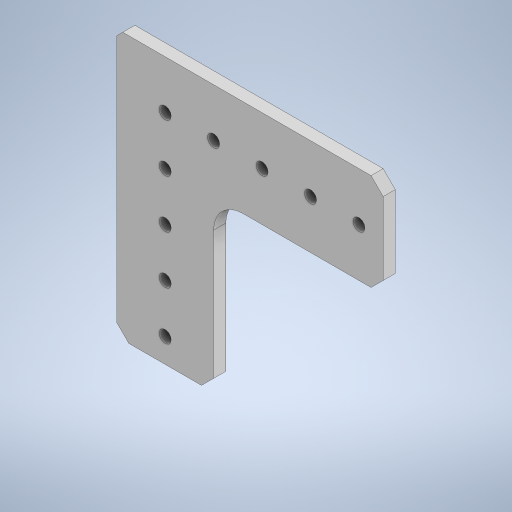
# Autodesk Inventor part: L-Bracket
Saved by Autodesk Inventor 2023 (Build 270158030, 158C)
## iProperties
Created: 2022-07-21
Part Number: L-Bracket
Material: Generic
Document SubType Name: Modeling
Designer: rm0990889
Density: 1 g/cm^3
Appearance: Default
Author: rm0990889
Autodesk Inventor part; units mm, degrees
ref_plane "YZ Plane" through (0, 0, 0) normal (1, 0, 0) x (0, 1, 0)
ref_plane "XZ Plane" through (0, 0, 0) normal (0, 1, 0) x (-1, 0, 0)
ref_plane "XY Plane" through (0, 0, 0) normal (0, 0, 1) x (1, 0, 0)
sketch "Sketch1" plane through (0, 0, 0) normal (0, 0, 1) x (1, 0, 0)
  circle A0 centre (12.7, -12.7) radius 1.5875
  line L0 (0, 0) -> (0, -14.9496)
  line L1 (0, 0) -> (27.0799, 0)
  circle A1 centre (25.4, -12.7) radius 1.5875
  circle A2 centre (38.1, -12.7) radius 1.5875
  circle A3 centre (50.8, -12.7) radius 1.5875
  circle A4 centre (63.5, -12.7) radius 1.5875
  circle A5 centre (12.7, -25.4) radius 1.5875
  circle A6 centre (12.7, -38.1) radius 1.5875
  circle A7 centre (12.7, -50.8) radius 1.5875
  circle A8 centre (12.7, -63.5) radius 1.5875
  line L2 (27.0799, 0) -> (66.675, 0)
  line L3 (69.85, -3.175) -> (69.85, -22.225)
  line L4 (0, -14.9496) -> (0, -66.675)
  line L5 (3.175, -69.85) -> (22.225, -69.85)
  line L6 (66.675, -25.4) -> (33.02, -25.4)
  line L7 (25.4, -33.02) -> (25.4, -66.675)
  arc A9 (33.02, -25.4) -> (25.4, -33.02) centre (33.02, -33.02) ccw
  line L8 (66.675, 0) -> (69.85, -3.175)
  line L9 (66.675, -25.4) -> (69.85, -22.225)
  line L10 (0, -66.675) -> (3.175, -69.85)
  line L11 (22.225, -69.85) -> (25.4, -66.675)
  line L12 (0, -1.5875) -> (1.5875, 0)
  point P0 (69.85, 0)
  point P1 (69.85, -25.4)
  point P2 (69.85, -12.7)
  point P3 (0, -69.85)
  point P4 (25.4, -69.85)
  dimension "d0" = 3.175
  dimension "d1" = 12.7
  dimension "d2" = 12.7
  dimension "d5" = 12.7
  dimension "d12" = 12.7
  dimension "d17" = 6.35
  dimension "d18" = 25.4
  dimension "d19" = 6.35
  dimension "d20" = 25.4
  dimension "d21" = 7.62
  dimension "d22" = 3.175
  dimension "d23" = 3.175
  dimension "d24" = 3.175
  dimension "d25" = 3.175
  dimension "d26" = 3.175
  dimension "d27" = 3.175
  dimension "d28" = 3.175
  dimension "d29" = 3.175
  constraints: 26 end point, 10 centre point, 10 point on line, 4 horizontal, 3 perpendicular, 3 vertical, 2 point on circle, 2 tangent, 1 midpoint, 16 other
  measures "d0" diameter of A0
  measures "d1" distance from line of A0.centre L1
  measures "d2" distance from line of A0.centre L0
  measures "d5" distance of A0.centre A1.centre
  measures "d12" distance of A0.centre A5.centre
  measures "d17" distance of point (69.85, -12.7) A4.centre
  measures "d18" distance of point (69.85, 0) point (69.85, -25.4)
  measures "d19" distance from line of L5 A8.centre
  measures "d20" distance of point (0, -69.85) point (25.4, -69.85)
  measures "d21" radius of A9
  measures "d22" distance of L2.end point (69.85, 0)
  measures "d23" distance of L3.start point (69.85, 0)
  measures "d24" distance of L6.start point (69.85, -25.4)
  measures "d25" distance of L3.end point (69.85, -25.4)
  measures "d26" distance of L4.end point (0, -69.85)
  measures "d27" distance of L5.start point (0, -69.85)
  measures "d28" distance of L5.end point (25.4, -69.85)
  measures "d29" distance of L7.end point (25.4, -69.85)
extrude "Extrusion1" add sketch "Sketch1" along normal blind 3.175 contours L12 L1 L2 L8 L3 L9 L6 A9 L7 L11 L5 L10 L4 L0
equation "\"d23\" = d22"
equation "\"d24\" = d22"
equation "\"d25\" = d24"
equation "\"d26\" = d22"
equation "\"d27\" = d26"
equation "\"d28\" = d22"
equation "\"d29\" = d28"
body "Solid1"
